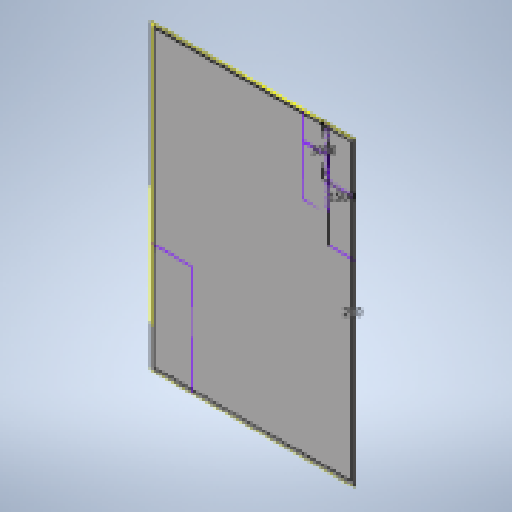
# Autodesk Inventor part: Part1
Saved by Autodesk Inventor 2026.2 (Build 302298000, 298)
## iProperties
Created: 2026-04-17
Part Number: Part1
Material: Generic
Document SubType Name: Sheet Metal
Designer: admin
Density: 1 g/cm^3
Sheet Metal Rule: Default_mm
Appearance: Default
Author: admin
Autodesk Inventor part; units mm, degrees
ref_plane "YZ Plane" through (0, 0, 0) normal (1, 0, 0) x (0, 1, 0)
ref_plane "XZ Plane" through (0, 0, 0) normal (0, 1, 0) x (-1, 0, 0)
ref_plane "XY Plane" through (0, 0, 0) normal (0, 0, 1) x (1, 0, 0)
sketch "Sketch1" plane through (0, 0, 0) normal (0, 0, 1) x (1, 0, 0)
  line L0 (6040, -8925) -> (-6040, -8925)
  line L1 (-6040, -8925) -> (-6040, 8925)
  line L2 (-6040, 8925) -> (6040, 8925)
  line L3 (6040, 8925) -> (6040, -8925)
  line L4 (6040, -8925) -> (-6040, 8925) construction
  line L5 (-6040, -8925) -> (6040, 8925) construction
  point P0 (0, 0)
  dimension "d0" = 12080
  dimension "d1" = 17850
  measures "d0" distance of L1.end L2.end
  measures "d1" distance of L0.end L1.end
extrude "Plate1" add sketch "Sketch1" along normal blind 6
sketch "Sketch2" plane through (0, 0, 6) normal (0, 0, 1) x (1, 0, 0)
  line L0 (6040, 8925) -> (6040, -8925)
  line L1 (-6040, 8925) -> (6040, 8925) projected
  line L2 (-6040, -8925) -> (-6040, 8925) projected
  line L3 (6040, -8925) -> (-6040, -8925) projected
  line L4 (5840, -8725) -> (5840, 8725)
  line L5 (5840, 8725) -> (-5840, 8725)
  line L6 (-5840, 8725) -> (-5840, -8725)
  line L7 (-5840, -8725) -> (5840, -8725)
  line L8 (6040, 8925) -> (-6040, 8925) projected
  line L9 (6040, 8925) -> (4540, 8925)
  line L10 (4540, 8925) -> (4540, 5925)
  line L11 (4540, 5925) -> (6040, 5925)
  line L12 (6040, 5925) -> (6040, 8925)
  line L13 (6040, -8925) -> (6040, 8925) projected
  line L14 (6040, 5915.3074) -> (4540, 5915.3074)
  line L15 (4540, 5915.3074) -> (4540, 2719.1164)
  line L16 (4540, 2719.1164) -> (6040, 2719.1164)
  line L17 (6040, 2719.1164) -> (6040, 5915.3074)
  line L18 (4480.7937, 7302.624) -> (2980.7937, 7302.624)
  line L19 (2980.7937, 7302.624) -> (2980.7937, 4345.2957)
  line L20 (2980.7937, 4345.2957) -> (4480.7937, 4345.2957)
  line L21 (4480.7937, 4345.2957) -> (4480.7937, 7302.624)
  line L22 (6040, 6064.5316) -> (4414.8344, 6064.5316) construction
  line L23 (4414.8344, 6064.5316) -> (4414.8344, 5939.4754) construction
  line L24 (4414.8344, 5939.4754) -> (6040, 5939.4754) construction
  line L25 (6040, 5939.4754) -> (6040, 6064.5316) construction
  line L26 (4414.8344, 5939.4754) -> (4552.3842, 5939.4754) construction
  line L27 (4552.3842, 5939.4754) -> (4552.3842, 4470.5931) construction
  line L28 (4552.3842, 4470.5931) -> (4414.8344, 4470.5931) construction
  line L29 (4414.8344, 4470.5931) -> (4414.8344, 5939.4754) construction
  line L30 (4521.5038, 8925) -> (3021.5038, 8925)
  line L31 (3021.5038, 8925) -> (3021.5038, 7257.6876)
  line L32 (3021.5038, 7257.6876) -> (4521.5038, 7257.6876)
  line L33 (4521.5038, 7257.6876) -> (4521.5038, 8925)
  line L34 (4548.1732, 8919.3279) -> (4414.8344, 8919.3279) construction
  line L35 (4414.8344, 8919.3279) -> (4414.8344, 6064.5316) construction
  line L36 (4414.8344, 6064.5316) -> (4548.1732, 6064.5316) construction
  line L37 (4548.1732, 6064.5316) -> (4548.1732, 8919.3279) construction
  line L38 (-6040, -8925) -> (-3545.5767, -8925)
  line L39 (-3545.5767, -8925) -> (-3545.5767, -2421.1359)
  line L40 (-3545.5767, -2421.1359) -> (-6040, -2421.1359)
  line L41 (-6040, -2421.1359) -> (-6040, -8925)
  dimension "d17" = 200
  dimension "d18" = 1500
  dimension "d19" = 3000
  constraints: 74 end point, 19 parallel, 8 horizontal, 8 perpendicular, 3 point on line, 3 other
  measures "d17" distance between parallel lines of L0 L4
  measures "d18" distance of L11.end L10.end
  measures "d19" distance of L10.end L9.end
equation "\"d2\" = Thickness"
equation "\"BendRadius\" = Thickness"
equation "\"BendReliefWidth\" = Thickness"
equation "\"BendReliefDepth\" = 0.5 * Thickness"
equation "\"CornerReliefSize\" = 4 * Thickness"
equation "\"MinimumRemnant\" = 2 * Thickness"
equation "\"TransitionRadius\" = BendRadius"
equation "\"JacobiRadiusSize\" = BendRadius"
equation "\"GapSize\" = Thickness"
equation "\"Thickness\" = 6"
body "Solid1"
